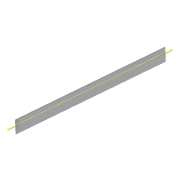
# Autodesk Inventor part: Scoring Platform
Saved by Autodesk Inventor 2015 (Build 190159000, 159)
## iProperties
Created: 2015-01-10
Part Number: Scoring Platform
Material: Generic
Document SubType Name: Modeling
Designer: Peter
Density: 1 g/cm^3
Appearance: Default
Author: Peter
Autodesk Inventor part; units mm, degrees
ref_plane "YZ Plane" through (0, 0, 0) normal (1, 0, 0) x (0, 1, 0)
ref_plane "XZ Plane" through (0, 0, 0) normal (0, 1, 0) x (-1, 0, 0)
ref_plane "XY Plane" through (0, 0, 0) normal (0, 0, 1) x (1, 0, 0)
sketch "Sketch1" plane through (0, 0, 0) normal (0, 0, 1) x (1, 0, 0)
  line L0 (0, 0) -> (-508, 0)
  line L1 (-508, 0) -> (-508, 4749.8)
  line L2 (-508, 4749.8) -> (0, 4749.8)
  line L3 (0, 4749.8) -> (0, 0)
  line L4 (0, 0) -> (-508, 0) construction
  dimension "width" = 508
  dimension "length" = 4749.8
  dimension "d2" = 508
  dimension "d3" = 508
  constraints: 10 end point, 3 horizontal, 2 parallel, 1 perpendicular, 1 vertical
  measures "width" distance of L0.start L0.end
  measures "length" distance of L2.end L0.start
  measures "d2" distance of L1.end L2.end
  measures "d3" distance of L0.start L4.end
ref_plane "Work Plane2" through (0, 4749.8, -49.8856) normal (0, 0, -1) x (0, -1, 0)
ref_plane "Work Plane1" through (0, 4749.8, 0) normal (0, 0, -1) x (0, -1, 0)
sketch "Sketch2" plane through (0, 4749.8, 0) normal (0, 0, -1) x (0, -1, 0)
  line L0 (4749.8, 0) -> (4749.8, 508) projected
  line L1 (0, 0) -> (4749.8, 0) projected
  line L2 (0, 508) -> (0, 0) projected
sketch "Sketch3" plane through (0, 4749.8, -49.8856) normal (0, 0, -1) x (0, -1, 0)
  line L0 (4749.8, 0) -> (4749.8, 508) projected
  line L1 (0, 0) -> (4749.8, 0) projected
  line L2 (4749.8, 508) -> (0, 508) projected
  line L3 (0, 508) -> (0, 0) projected
  line L4 (-10.9008, 518.9008) -> (4760.7008, 518.9008)
  line L5 (4760.7008, 518.9008) -> (4760.7008, -10.9008)
  line L6 (4760.7008, -10.9008) -> (-10.9008, -10.9008)
  line L7 (-10.9008, -10.9008) -> (-10.9008, 518.9008)
  line L8 (-173.9646, 681.9646) -> (4923.7646, 681.9646)
  line L9 (4923.7646, 681.9646) -> (4923.7646, -173.9646)
  line L10 (4923.7646, -173.9646) -> (-173.9646, -173.9646)
  line L11 (-173.9646, -173.9646) -> (-173.9646, 681.9646)
  dimension "d5" = 855.9292
  dimension "d6" = 5097.7292
  constraints: 16 end point, 6 other
  measures "d5" distance of L8.end L9.end
  measures "d6" distance of L8.start L8.end
loft "Loft1" add profiles "Sketch1", "Sketch3" contours all / L1 L3 L2 L0 | L4 L5 L6 L7 | L8 L9 L10 L11
ref_plane "Work Plane3" through (-254, -173.9646, 72.8363) normal (1, 0, 0) x (0, 1, 0)
body "Solid1"
